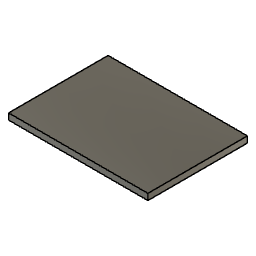
final assembly v2 (Autodesk Fusion 360 archive; units mm, degrees)
design "cover"
Autodesk Fusion 360 part; units mm, degrees
sketch "Sketch1" plane through (0, 0, 0) normal (0, 0, 1) x (1, 0, 0)
  line L0 (0, 0) -> (-71.12, 0)
  line L1 (-71.12, 0) -> (-71.12, 50.8)
  line L2 (-71.12, 50.8) -> (0, 50.8)
  line L3 (0, 50.8) -> (0, 0)
  dimension "d1" = 71.12
  dimension "d2" = 50.8
  constraint horizontal L0
  constraint vertical L1
  constraint horizontal L2
  constraint vertical L3
  constraint coincident L0.start L3.end
  measures "d1" distance of L0.start L0.end
  measures "d2" distance of L0.start L2.end
extrude "Extrude1" add sketch "Sketch1" along normal blind 3.175
component "Component" placed x (1, 0, 0) y (0, 1, 0) z (0, 0, 1) at (0, 0, 0)
equation "d1 = 3 in - 0.2 in"

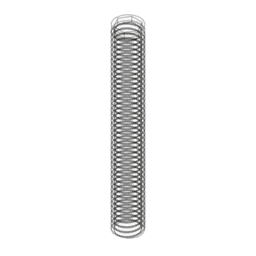
design "bolts"
Autodesk Fusion 360 part; units mm, degrees
sketch "Sketch1" plane through (0, 0, 0) normal (0, 0, 1) x (1, 0, 0)
  circle A0 centre (0, 0) radius 6.35
  dimension "d1" = 12.7
  constraint coincident A0.centre origin
  measures "d1" diameter of A0
extrude "Extrude1" add sketch "Sketch1" along normal blind 88.9
thread "Thread1" "Custom Threads 0.5 1/2-12 UNS 3A" major diameter 11.9275 minor diameter 9.6713 pitch 2.1167 angle 60 modelled right hand crest width 0.3562 on face at (6.3421, -0.3165, 59.2667) from (0, 0, 0) to (0, 0, 86.36) crest through (5.9637, 0, -0.5292)
sketch "Sketch2" plane through (0, 0, 88.9) normal (0, 0, 1) x (-1, 0, 0)
  line L0 (-2.5875, -4.4817) -> (-5.175, 0)
  line L1 (-5.175, 0) -> (-2.5875, 4.4817)
  line L2 (-2.5875, 4.4817) -> (2.5875, 4.4817)
  line L3 (2.5875, 4.4817) -> (5.175, 0)
  line L4 (5.175, 0) -> (2.5875, -4.4817)
  line L5 (2.5875, -4.4817) -> (-2.5875, -4.4817)
  line L6 (-5.175, 0) -> (5.175, 0) construction
  circle A0 centre (0, 0) radius 5.9637
  line L7 (0, 0) -> (0, -5.9637) construction
  line L8 (0, 0) -> (0, 5.9637) construction
  line L9 (0, 0) -> (-5.9637, 0) construction
  line L10 (0, 0) -> (5.9637, 0) construction
  line L11 (-2.5875, 4.4817) -> (-2.5875, -4.4817) construction
  dimension "d6" = 120
  dimension "d7" = 120
  dimension "d8" = 120
  dimension "d9" = 10.35
  constraint equal L0 L1
  constraint equal L1 L2
  constraint equal L2 L3
  constraint equal L3 L4
  constraint equal L4 L5
  constraint midpoint L6 A0.centre
  constraint coincident A0.centre L7.start
  constraint coincident A0 L7.end
  constraint vertical L7
  constraint coincident A0 L8.end
  constraint vertical L8
  constraint equal L7 L8
  constraint coincident A0 L9.end
  constraint horizontal L9
  constraint coincident A0 L10.end
  constraint parallel L9 L10
  constraint equal L9 L10
  constraint horizontal L5
  measures "d6" angle of L0 L5
  measures "d7" angle of L0 L1
  measures "d8" angle of L1 L2
  measures "d9" horizontal distance of L0.end L3.end
extrude "Extrude2" cut sketch "Sketch2" against normal blind 2.54 contours L0 L1 L2 L3 L4 L5
component "Component" placed x (1, 0, 0) y (0, 1, 0) z (0, 0, 1) at (0, 0, 0)
equation "d9 = ( 1 / 4 ) * 1 in + 4 mm"
